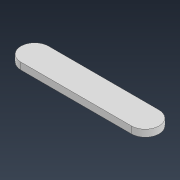
# Autodesk Inventor part: Phone Stand Bump
Saved by Autodesk Inventor 2021 (Build 250183000, 183)
## iProperties
Created: 2021-01-30
Part Number: Phone Stand Bump
Material: Generic
Document SubType Name: Modeling
Designer: PaisW
Density: 1 g/cm^3
Appearance: Default
Author: PaisW
Autodesk Inventor part; units mm, degrees
ref_plane "YZ Plane" through (0, 0, 0) normal (1, 0, 0) x (0, 1, 0)
ref_plane "XZ Plane" through (0, 0, 0) normal (0, 1, 0) x (-1, 0, 0)
ref_plane "XY Plane" through (0, 0, 0) normal (0, 0, 1) x (1, 0, 0)
sketch "Sketch1" plane through (0, 0, 0) normal (0, 1, 0) x (-1, 0, 0)
  line L0 (40, -10) -> (-40, -10)
  arc A0 (-40, 10) -> (-40, -10) centre (-40, 0) ccw
  line L1 (-40, 10) -> (40, 10)
  arc A1 (40, -10) -> (40, 10) centre (40, 0) ccw
  point P0 (0, 0)
  point P1 (0, -10)
  point P2 (-50, 0)
  dimension "d0" = 10
  dimension "d1" = 80
  constraints: 5 point on circle, 4 end point, 4 tangent, 2 centre point, 2 horizontal, 1 horizontal alignment, 1 midpoint, 1 vertical alignment
  measures "d0" radius of A0
  measures "d1" distance of A0.centre A1.centre
extrude "Extrusion1" add sketch "Sketch1" along normal blind 5
body "Solid1"
